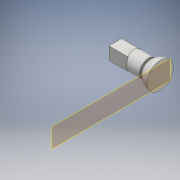
# Autodesk Inventor part: soportebrazo
Saved by Autodesk Inventor 2016 (Build 200138000, 138)
## iProperties
Created: 2016-02-20
Part Number: soportebrazo
Material: Genérico
Document SubType Name: Modeling
Designer: Usuario1
Density: 1 g/cm^3
Appearance: Valor por defecto
Author: Usuario1
Autodesk Inventor part; units mm, degrees
ref_plane "XZ Plane" through (0, 0, 0) normal (0, 1, 0) x (-1, 0, 0)
ref_plane "XY Plane" through (0, 0, 0) normal (0, 0, 1) x (1, 0, 0)
sketch "Boceto1" plane through (0, 0, 0) normal (1, 0, 0) x (0, 1, 0)
  line L0 (1.0744, 1.2847) -> (7.0094, 1.2847)
  line L1 (1.1029, 0.9847) -> (6.9809, 0.9847)
  arc A0 (1.0744, 1.2847) -> (0, 0) centre (1.3052, 0) ccw
  arc A1 (1.1029, 0.9847) -> (0.3, 0) centre (1.3052, 0) ccw
  arc A2 (8.0838, 0) -> (7.0094, 1.2847) centre (6.7786, 0) ccw
  arc A3 (7.7838, 0) -> (6.9809, 0.9847) centre (6.7786, 0) ccw
  line L2 (6.7094, 0.4) -> (6.7094, -0.4)
  line L3 (5.9094, -0.4) -> (5.9094, 0.4)
  line L4 (0.3, 0) -> (0, 0)
  line L5 (7.7838, 0) -> (8.0838, 0)
  circle A4 centre (1.3052, 0) radius 0.45
  line L6 (6.7094, 0.4) -> (5.9094, 0.4)
  line L7 (6.7094, -0.4) -> (5.9094, -0.4)
  point P0 (0, 0)
  constraints: 16 end point, 8 point on circle, 5 centre point
extrude "Extrusión1" add sketch "Boceto1" along normal blind 2.1095 contours L2 L7 L3 L6
sketch "Boceto2" plane through (2.1095, 0, 0) normal (1, 0, 0) x (0, 0, -1)
  line L0 (0.4, 6.7094) -> (-0.4, 6.7094) projected
  line L1 (-0.4, 6.7094) -> (-0.4, 5.9094) projected
  line L2 (-0.4, 5.9094) -> (0.4, 5.9094) projected
  line L3 (0.4, 5.9094) -> (0.4, 6.7094) projected
  line L4 (0.4, 6.7094) -> (-0.4, 6.7094) projected
  line L5 (-0.4, 6.7094) -> (-0.4, 5.9094) projected
  circle A0 centre (0, 6.3094) radius 0.5657
  point P0 (0, 0)
  constraints: 3 other
extrude "Extrusión2" add sketch "Boceto2" against normal blind 2.1095 contours A0 L3 | L0 A0 | L1 A0 | A0 L2
sketch "Boceto3" plane through (0, 0, 0) normal (1, 0, 0) x (0, 1, 0)
  line L0 (1.0744, 1.2847) -> (7.0094, 1.2847)
  line L1 (1.1029, 0.9847) -> (6.9809, 0.9847)
  arc A0 (1.0744, 1.2847) -> (0, 0) centre (1.3052, 0) ccw
  arc A1 (1.1029, 0.9847) -> (0.3, 0) centre (1.3052, 0) ccw
  arc A2 (8.0838, 0) -> (7.0094, 1.2847) centre (6.7786, 0) ccw
  arc A3 (7.7838, 0) -> (6.9809, 0.9847) centre (6.7786, 0) ccw
  line L2 (0.3, 0) -> (0, 0)
  line L3 (7.7838, 0) -> (8.0838, 0)
  line L4 (7.7838, 0) -> (0.3, 0)
  point P0 (0, 0)
  constraints: 10 end point, 8 point on circle, 4 centre point, 1 horizontal
revolve "Revolución1" cut sketch "Boceto3" angle 360 about axis through (0, 7.7838, 0) along (0, -1, 0)
sketch "Boceto4" plane through (0, 0, 0) normal (1, 0, 0) x (0, 1, 0)
  line L0 (1.0744, 1.2847) -> (7.0094, 1.2847)
  line L1 (1.1029, 0.9847) -> (6.9809, 0.9847)
  arc A0 (1.0744, 1.2847) -> (0, 0) centre (1.3052, 0) ccw
  arc A1 (1.1029, 0.9847) -> (0.3, 0) centre (1.3052, 0) ccw
  arc A2 (8.0838, 0) -> (7.0094, 1.2847) centre (6.7786, 0) ccw
  arc A3 (7.7838, 0) -> (6.9809, 0.9847) centre (6.7786, 0) ccw
  line L2 (6.7094, 0.4) -> (6.7094, -0.4)
  line L3 (5.9094, -0.4) -> (5.9094, 0.4)
  line L4 (0.3, 0) -> (0, 0)
  line L5 (7.7838, 0) -> (8.0838, 0)
  circle A4 centre (1.3052, 0) radius 0.45
  line L6 (6.7094, 0.4) -> (5.9094, 0.4)
  line L7 (6.7094, -0.4) -> (5.9094, -0.4)
  point P0 (0, 0)
  constraints: 16 end point, 8 point on circle, 5 centre point
extrude "Extrusión3" add sketch "Boceto4" along normal blind 2.1095 contours L2 L7 L3 L6
ref_plane "Plano de trabajo1" through (2.8443, 0, 0) normal (1, 0, 0) x (0, 1, 0)
sketch "Boceto5" plane through (2.8443, 0, 0) normal (1, 0, 0) x (0, 1, 0)
  circle A0 centre (6.3094, 0) radius 0.5657 projected
  line L0 (7.146, 0) -> (5.4727, 0)
  arc A1 (7.146, 0) -> (5.4727, 0) centre (6.3094, 0) ccw
  point P0 (0, 0)
  constraints: 2 end point, 2 point on circle, 1 centre point, 1 horizontal
revolve "Revolución2" add sketch "Boceto5" angle 180 about axis through (2.8443, 7.146, 0) along (0, -1, 0) picked at (6.4505, 0.2153) contours L0 A0 | A0 L0 A1
